WP 3385088 Upper Rack Wheel (8258787 or 8258787G) (Autodesk Fusion 360 design; units mm, degrees)
Autodesk Fusion 360 part; units mm, degrees
note: some values were not read from the file. Set by a fixed rule: which sketch regions a step uses.
sketch "Sketch2" plane through (0, 0, 0) normal (0, 1, 0) x (1, 0, 0)
  line L0 (6.35, -15.0812) -> (9.1281, -15.0812)
  line L1 (9.1281, -15.0812) -> (9.1281, -3.175)
  line L2 (9.1281, -3.175) -> (13.6922, -3.175)
  line L3 (15.2797, -1.5875) -> (15.2797, 0.3969)
  arc A0 (15.2797, 0.3969) -> (14.4859, 1.1906) centre (14.4859, 0.3969) ccw
  line L4 (14.4859, 1.1906) -> (13.8906, 1.1906)
  arc A1 (13.8906, 1.1906) -> (12.3031, -0.3969) centre (13.8906, -0.3969) ccw
  line L5 (12.3031, -0.3969) -> (7.4613, -0.3969)
  line L6 (7.4613, -0.3969) -> (7.4613, -2.0638)
  line L7 (7.4613, -2.0638) -> (6.35, -3.175)
  line L8 (6.35, -3.175) -> (6.35, -15.0812)
  line L9 (13.6922, -3.175) -> (15.2797, -1.5875)
  dimension "d14" = 135
  dimension "d17" = 11.9062
  dimension "d18" = 14.6844
  dimension "d19" = 11.9062
  dimension "d20" = 9.1281
  dimension "d21" = 6.35
  dimension "d22" = 7.4612
  dimension "d23" = 1.6669
  dimension "d24" = 135
  dimension "d26" = 0.7937
  dimension "d27" = 15.2797
  dimension "d28" = 4.3656
  dimension "d29" = 12.3031
  dimension "d30" = 1.5875
  constraint horizontal L0
  constraint perpendicular L0 L1
  constraint perpendicular L1 L2
  constraint perpendicular L2 L3
  constraint tangent L3 A0
  constraint perpendicular L3 L4
  constraint tangent L4 A1
  constraint horizontal L5
  constraint perpendicular L5 L6
  constraint parallel L1 L8
  constraint coincident L0.start L8.end
  constraint tangent A0 L4
  constraint coincident A1.centre L5
  measures "d14" angle of L6 L7
  measures "d17" distance of L7.end L0.start
  measures "d18" distance of L0 L5
  measures "d19" distance of L0 L2
  measures "d20" horizontal distance of L0.end origin
  measures "d21" distance of L8 origin
  measures "d22" distance of L6 origin
  measures "d23" distance of L5.end L6.end
  measures "d24" angle of L2 L9
  measures "d26" radius of A0
  measures "d27" distance of L3 origin
  measures "d28" distance of L2 L4
  measures "d29" horizontal distance of A1.end origin
  measures "d30" vertical distance of L2.end L3.start
revolve "Revolve1" add sketch "Sketch2" angle 360 about axis through (0, 0, 1.75) along (0, 0, 1)
equation "d14 = 180 deg - 45 deg"
equation "d17 = ( 15 / 32 ) * 1 in"
equation "d18 = ( 18.5 / 32 ) * 1 in"
equation "d19 = ( 15 / 32 ) * 1 in"
equation "d20 = ( 23 / 64 ) * 1 in"
equation "d21 = ( 16 / 64 ) * 1 in"
equation "d22 = ( 18.8 / 64 ) * 1 in"
equation "d26 = ( 2 / 64 ) * 1 in"
equation "d27 = ( 38.5 / 64 ) * 1 in"
equation "d28 = ( 5.5 / 32 ) * 1 in"
equation "d29 = ( 31 / 64 ) * 1 in"
equation "d30 = ( 2 / 32 ) * 1 in"
